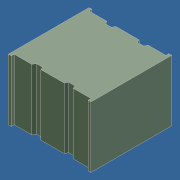
# Autodesk Inventor part: M20_ang2830TX-switch
Saved by Autodesk Inventor 2014 (Build 180170000, 170)
## iProperties
Category: PARTsolutions
Created: 2013-12-29
Part Number: M20_ang2830TX-switch
Catalog Web Link: www.cadenas.de
Description: Angle Mount Miniature Rockers- Switch - Series M - Miniature Rockers
Document SubType Name: Modeling
Designer: PARTsolutions
Material: Generic
Density: 1 g/cm^3
Appearance: RGB(78,110,71)
PSOL_NOTUSEDSKLST: SKLST{SKETCH{NAME{"Sketch 1"}MAT{1,0,0,0,0,0,-1,0,0,1,0,0,0,-0.3777,0,1}SKETCHON{PLANE{"Reference plane 2"}}LOOP{LINE{POINT{-0.21333333333333,0.18006518518519}POINT{-0.21333333333333,-0.18006518518519}}ARC{POINT{-0.21333333333333,-0.18006518518519}POINT{-0.21183372005301,-0.18368557190486}POINT{-0.20821333333333,-0.18518518518519}}LINE{POINT{-0.20821333333333,-0.18518518518519}POINT{0.20821333333333,-0.18518518518519}}ARC{POINT{0.20821333333333,-0.18518518518519}POINT{0.21183372005301,-0.18368557190486}POINT{0.21333333333333,-0.18006518518519}}LINE{POINT{0.21333333333333,-0.18006518518519}POINT{0.21333333333333,0.18006518518519}}ARC{POINT{0.21333333333333,0.18006518518519}POINT{0.21183372005301,0.18368557190486}POINT{0.20821333333333,0.18518518518519}}LINE{POINT{0.20821333333333,0.18518518518519}POINT{-0.20821333333333,0.18518518518519}}ARC{POINT{-0.20821333333333,0.18518518518519}POINT{-0.21183372005301,0.18368557190486}POINT{-0.21333333333333,0.18006518518519}}}}SKETCH{NAME{"Sketch 7"}MAT{1,0,0,0,0,0,-1,0,0,1,0,0,0,-0.3777,0,1}SKETCHON{PLANE{"Reference plane 2"}}LOOP{LINE{POINT{-0.2,-0.11}POINT{-0.17,-0.11}}LINE{POINT{-0.17,-0.11}POINT{-0.17,-0.04}}LINE{POINT{-0.17,-0.04}POINT{-0.2,-0.04}}LINE{POINT{-0.2,-0.04}POINT{-0.2,-0.11}}}}}
NB: M20_ang2830TX-switch
NN: Angle Mount Miniature Rockers- Switch
NT: Series M - Miniature Rockers
NBSYN: $PN.-switch
LINA: M20_ang2830TX-switch
PN: M20_ang2830TX
SRS: M20
PLS: 2
CRCTSALG: '2','2 - ON/NONE/ON','3','3 - ON/OFF/ON','5','5 - ON/NONE/(ON)','8','8 - (ON)/OFF/(ON)','9','9 - ON/OFF/(ON)','4', '4 - ON/ON/ON','6','6 - (ON)/ON/(ON)','7','7 - ON/ON/(ON)'
CRCTS: 8
FRMALG: 'TX', 'TX - Narrow Frame for Small Actuator', 'TZ'  , 'TZ - Wide Frame for Large Actuator'
FRM: TX
TRMNLSALG: '30','30 - .150" (3.81mm) Right Angle PC (1-3 Pole)', '40','40 - .150" (3.81mm) Vertical PC (1-4 Pole)','45', '45 - .100" (2.54mm) Vertical PC (1-4 Pole)'
TRMNLS: 30
WIDTH: 0.512
HEIGHT: 0.388
LENGTH: 0.500
A: 0.150
TRMNLNOH: 2.000
TRMNLOV: 3.000
LTRMNL: 0.031
POS: 0.075
POS2: 0.185
POS3: 0.150
D: 0.075
HOLES: 0.185
WH: 0.15000
D1: 0.00000
D2: 0.07500
KT: DUMMY
SUPPLIER: NKKSWITCHES
ARTICLENO: M20_ang2830TX-switch
BOMINFO: M20_ang2830TX-switch
CREATOR: CADENAS GmbH
PSOL_IDENT_0: {$CADENAS_DATA\23d-libs\nkkswitches\toggle\m\parts\m_ang_t_switch.prj},233 {VTYP=3D},{NB=M20_ang2830
PSOL_IDENT_1: TX-switch},{LINA=M20_ang2830TX-switch},{NN=Angle Mount Miniature Rockers- Switch},{DATE=28.05.2007 0
PSOL_IDENT_2: 7:42:30},{GEOMDATE=28.05.2007 07:37:00},{VERSION=},{LINEID=10},{LINESUBID=-1},{WBVAR=PLS,CRCTS,FRM,T
PSOL_IDENT_3: RMNLS}  {NB=M20_ang2830TX-switch},{LINA=M20_ang2830TX-switch},{KT=DUMMY},{PN=M20_ang2830TX},{SRS=M20
PSOL_IDENT_4: },{PLS=2},{CRCTSALG='2','2 - ON/NONE/ON','3','3 - ON/OFF/ON','5','5 - ON/NONE/(ON)','8','8 - (ON)/OF
PSOL_IDENT_5: F/(ON)','9','9 - ON/OFF/(ON)','4', '4 - ON/ON/ON','6','6 - (ON)/ON/(ON)','7','7 - ON/ON/(ON)'},{CRCT
PSOL_IDENT_6: S=8},{FRMALG='TX', 'TX - Narrow Frame for Small Actuator', 'TZ'  , 'TZ - Wide Frame for Large Actuat
PSOL_IDENT_7: or'},{FRM=TX},{TRMNLSALG='30','30 - .150\" (3.81mm) Right Angle PC (1-3 Pole)', '40','40 - .150\" (3
PSOL_IDENT_8: .81mm) Vertical PC (1-4 Pole)','45', '45 - .100\" (2.54mm) Vertical PC (1-4 Pole)'},{TRMNLS=30},{WID
PSOL_IDENT_9: TH=0.512},{HEIGHT=0.3877},{LENGTH=0.5},{A=0.15},{TRMNLNOH=2},{TRMNLOV=3},{LTRMNL=0.031},{POS=0.075},
PSOL_IDENT_10: {POS2=0.185},{POS3=0.15},{D=0.075},{HOLES=0.185},{WH=0.15000},{D1=0.00000},{D2=0.07500}
Title: M20_ang2830TX-switch
Author: Cadenas PARTsolutions
Comments: Series M - Miniature Rockers
Autodesk Inventor part; units mm, degrees
sketch "Sketch_2" plane through (0, -0.254, 0) normal (0, 1, 0) x (1, 0, 0)
  line L0 (-6.5024, -6.35) -> (-6.0389, -6.35)
  line L1 (-6.0389, -6.35) -> (-6.0389, -5.8865)
  line L2 (-6.0389, -5.8865) -> (-3.2509, -5.8865)
  line L3 (-3.2509, -5.8865) -> (-3.0348, -5.4229)
  line L4 (-3.0348, -5.4229) -> (-2.0452, -5.4229)
  line L5 (-2.0452, -5.4229) -> (-1.8291, -5.8865)
  line L6 (-1.8291, -5.8865) -> (1.8291, -5.8865)
  line L7 (1.8291, -5.8865) -> (2.0452, -5.4229)
  line L8 (2.0452, -5.4229) -> (3.0348, -5.4229)
  line L9 (3.0348, -5.4229) -> (3.2509, -5.8865)
  line L10 (3.2509, -5.8865) -> (6.0389, -5.8865)
  line L11 (6.0389, -5.8865) -> (6.0389, -6.35)
  line L12 (6.0389, -6.35) -> (6.5024, -6.35)
  line L13 (6.5024, -6.35) -> (6.5024, 6.35)
  line L14 (6.5024, 6.35) -> (6.0389, 6.35)
  line L15 (6.0389, 6.35) -> (6.0389, 5.8865)
  line L16 (6.0389, 5.8865) -> (3.2509, 5.8865)
  line L17 (3.2509, 5.8865) -> (3.0348, 5.4229)
  line L18 (3.0348, 5.4229) -> (2.0452, 5.4229)
  line L19 (2.0452, 5.4229) -> (1.8291, 5.8865)
  line L20 (1.8291, 5.8865) -> (-1.8291, 5.8865)
  line L21 (-1.8291, 5.8865) -> (-2.0452, 5.4229)
  line L22 (-2.0452, 5.4229) -> (-3.0348, 5.4229)
  line L23 (-3.0348, 5.4229) -> (-3.2509, 5.8865)
  line L24 (-3.2509, 5.8865) -> (-6.0389, 5.8865)
  line L25 (-6.0389, 5.8865) -> (-6.0389, 6.35)
  line L26 (-6.0389, 6.35) -> (-6.5024, 6.35)
  line L27 (-6.5024, 6.35) -> (-6.5024, -6.35)
  constraints: 56 end point
extrude "Extrusion1" add sketch "Sketch_2" against normal blind 9.8476
sketch "Sketch_8" plane through (0, -9.5936, 0) normal (0, 1, 0) x (1, 0, 0)
  line L0 (-5.08, -2.794) -> (-4.318, -2.794)
  line L1 (-4.318, -2.794) -> (-4.318, -1.016)
  line L2 (-4.318, -1.016) -> (-5.08, -1.016)
  line L3 (-5.08, -1.016) -> (-5.08, -2.794)
  constraints: 8 end point
extrude "Extrusion2" cut sketch "Sketch_8" against normal blind 25.4
sketch "Sketch_5" plane through (0, -9.5936, 0) normal (0, 1, 0) x (1, 0, 0)
  line L0 (-0.381, -2.794) -> (0.381, -2.794)
  line L1 (0.381, -2.794) -> (0.381, -1.016)
  line L2 (0.381, -1.016) -> (-0.381, -1.016)
  line L3 (-0.381, -1.016) -> (-0.381, -2.794)
  constraints: 8 end point
extrude "Extrusion3" cut sketch "Sketch_5" against normal blind 25.4
sketch "Sketch_9" plane through (0, -9.5936, 0) normal (0, 1, 0) x (1, 0, 0)
  line L0 (4.318, -2.794) -> (5.08, -2.794)
  line L1 (5.08, -2.794) -> (5.08, -1.016)
  line L2 (5.08, -1.016) -> (4.318, -1.016)
  line L3 (4.318, -1.016) -> (4.318, -2.794)
  constraints: 8 end point
extrude "Extrusion4" cut sketch "Sketch_9" against normal blind 25.4
sketch "Sketch_10" plane through (0, -9.5936, 0) normal (0, 1, 0) x (1, 0, 0)
  line L0 (-5.08, 1.016) -> (-4.318, 1.016)
  line L1 (-4.318, 1.016) -> (-4.318, 2.794)
  line L2 (-4.318, 2.794) -> (-5.08, 2.794)
  line L3 (-5.08, 2.794) -> (-5.08, 1.016)
  constraints: 8 end point
extrude "Extrusion5" cut sketch "Sketch_10" against normal blind 25.4
sketch "Sketch_11" plane through (0, -9.5936, 0) normal (0, 1, 0) x (1, 0, 0)
  line L0 (-0.381, 1.016) -> (0.381, 1.016)
  line L1 (0.381, 1.016) -> (0.381, 2.794)
  line L2 (0.381, 2.794) -> (-0.381, 2.794)
  line L3 (-0.381, 2.794) -> (-0.381, 1.016)
  constraints: 8 end point
extrude "Extrusion6" cut sketch "Sketch_11" against normal blind 25.4
sketch "Sketch_12" plane through (0, -9.5936, 0) normal (0, 1, 0) x (1, 0, 0)
  line L0 (4.318, 1.016) -> (5.08, 1.016)
  line L1 (5.08, 1.016) -> (5.08, 2.794)
  line L2 (5.08, 2.794) -> (4.318, 2.794)
  line L3 (4.318, 2.794) -> (4.318, 1.016)
  constraints: 8 end point
extrude "Extrusion7" cut sketch "Sketch_12" against normal blind 25.4
sketch "Sketch_19" plane through (0, -0.254, 0) normal (0, 1, 0) x (1, 0, 0)
  line L0 (-6.5024, -6.35) -> (-6.0389, -6.35)
  line L1 (-6.0389, -6.35) -> (-6.0389, -5.8865)
  line L2 (-6.0389, -5.8865) -> (-3.2509, -5.8865)
  line L3 (-3.2509, -5.8865) -> (-3.0348, -5.4229)
  line L4 (-3.0348, -5.4229) -> (-2.0452, -5.4229)
  line L5 (-2.0452, -5.4229) -> (-1.8291, -5.8865)
  line L6 (-1.8291, -5.8865) -> (1.8291, -5.8865)
  line L7 (1.8291, -5.8865) -> (2.0452, -5.4229)
  line L8 (2.0452, -5.4229) -> (3.0348, -5.4229)
  line L9 (3.0348, -5.4229) -> (3.2509, -5.8865)
  line L10 (3.2509, -5.8865) -> (6.0389, -5.8865)
  line L11 (6.0389, -5.8865) -> (6.0389, -6.35)
  line L12 (6.0389, -6.35) -> (6.5024, -6.35)
  line L13 (6.5024, -6.35) -> (6.5024, 6.35)
  line L14 (6.5024, 6.35) -> (6.0389, 6.35)
  line L15 (6.0389, 6.35) -> (6.0389, 5.8865)
  line L16 (6.0389, 5.8865) -> (3.2509, 5.8865)
  line L17 (3.2509, 5.8865) -> (3.0348, 5.4229)
  line L18 (3.0348, 5.4229) -> (2.0452, 5.4229)
  line L19 (2.0452, 5.4229) -> (1.8291, 5.8865)
  line L20 (1.8291, 5.8865) -> (-1.8291, 5.8865)
  line L21 (-1.8291, 5.8865) -> (-2.0452, 5.4229)
  line L22 (-2.0452, 5.4229) -> (-3.0348, 5.4229)
  line L23 (-3.0348, 5.4229) -> (-3.2509, 5.8865)
  line L24 (-3.2509, 5.8865) -> (-6.0389, 5.8865)
  line L25 (-6.0389, 5.8865) -> (-6.0389, 6.35)
  line L26 (-6.0389, 6.35) -> (-6.5024, 6.35)
  line L27 (-6.5024, 6.35) -> (-6.5024, -6.35)
  constraints: 56 end point
extrude "Extrusion8" cut sketch "Sketch_19" against normal blind 0.254
ref_plane "rot_XY" through (0, 6.6675, 0) normal (0, 0, 1) x (1, 0, 0)
ref_plane "rot_YZ" through (0, 6.6675, 0) normal (1, 0, 0) x (0, 1, 0)
ref_plane "rot_ZX" through (0, 6.6675, 0) normal (0, 1, 0) x (0, 0, 1)
ref_plane "to_cover_XY" through (0, -0.254, 0) normal (0, 1, 0) x (1, 0, 0)
ref_plane "to_cover_YZ" through (0, -0.254, 0) normal (1, 0, 0) x (0, 0, -1)
ref_plane "to_cover_ZX" through (0, -0.254, 0) normal (0, 0, -1) x (0, 1, 0)
ref_plane "to_terminals_XY" through (0, -9.5936, 0) normal (0, -1, 0) x (1, 0, 0)
ref_plane "to_terminals_YZ" through (0, -9.5936, 0) normal (1, 0, 0) x (0, 0, 1)
ref_plane "to_terminals_ZX" through (0, -9.5936, 0) normal (0, 0, 1) x (0, -1, 0)
body "Solid1"
